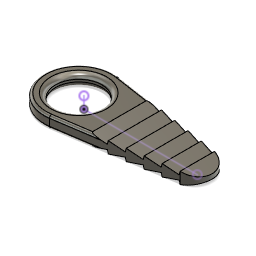
ZugPropfen (Autodesk Fusion 360 design; units mm, degrees)
Autodesk Fusion 360 part; units mm, degrees
sketch "Skizze1" plane through (0, 0, 0) normal (0, 1, 0) x (1, 0, 0)
  circle A0 centre (0, 0) radius 10
  circle A1 centre (0, 0) radius 15
  circle A2 centre (50, 0) radius 7.5
  line L0 (2.25, 14.8303) -> (51.125, 7.4151)
  line L1 (51.125, -7.4151) -> (2.25, -14.8303)
  dimension "d1" = 20
  dimension "d2" = 5
  dimension "d3" = 15
  dimension "d5" = 50
  constraint coincident A0.centre A1.centre
  constraint concentric A0 A1
  constraint coincident A1 L0.start
  constraint coincident A2 L0.end
  constraint tangent A2 L0
  constraint coincident A2 L1.start
  constraint coincident A1 L1.end
  constraint tangent A1 L1
  constraint tangent A1 L0
  constraint tangent A2 L1
  constraint horizontal A0.centre A2.centre
  measures "d1" diameter of A0
  measures "d2" distance of A0 A1
  measures "d3" diameter of A2
  measures "d5" distance of A0.centre A2.centre
extrude "Extrusion1" add sketch "Skizze1" along normal mid plane 5
sketch "Skizze2" plane through (0, 0, 0) normal (0, 0, 1) x (1, 0, 0)
  line L0 (2.25, 2.5) -> (2.25, -2.5)
  line L1 (2.25, -2.5) -> (51.125, -2.5)
sketch "Skizze3" plane through (0, 0, 0) normal (0, 0, 1) x (1, 0, 0)
  line L0 (17.5, 2.5) -> (57.5, 2.5)
  line L1 (57.5, 2.5) -> (57.5, 1)
  line L2 (57.5, 1) -> (51.1276, 2.5)
  line L3 (51.1276, 2.5) -> (50.7745, 1)
  line L4 (50.7745, 1) -> (44.4021, 2.5)
  line L5 (44.4021, 2.5) -> (44.049, 1)
  line L6 (44.049, 1) -> (37.6765, 2.5)
  line L7 (37.6765, 2.5) -> (37.3235, 1)
  line L8 (37.3235, 1) -> (30.951, 2.5)
  line L9 (30.951, 2.5) -> (30.5979, 1)
  line L10 (30.5979, 1) -> (24.2255, 2.5)
  line L11 (24.2255, 2.5) -> (23.8724, 1)
  line L12 (23.8724, 1) -> (17.5, 2.5)
  line L13 (23.8724, 1) -> (57.5, 1) construction
  line L14 (24.2255, 2.5) -> (51.1276, 2.5) construction
  line L15 (51.125, -2.5) -> (51.125, 2.5)
  line L16 (2.25, 2.5) -> (51.125, 2.5)
  line L17 (1.75, 0) -> (22.5, 0)
  line L18 (44.049, -1) -> (37.6765, -2.5)
  line L19 (23.8724, -1) -> (17.5, -2.5)
  line L20 (17.5, -2.5) -> (57.5, -2.5)
  line L21 (24.2255, -2.5) -> (23.8724, -1)
  line L22 (30.951, -2.5) -> (30.5979, -1)
  line L23 (51.1276, -2.5) -> (50.7745, -1)
  line L24 (37.3235, -1) -> (30.951, -2.5)
  line L25 (23.8724, -1) -> (57.5, -1) construction
  line L26 (24.2255, -2.5) -> (51.1276, -2.5) construction
  line L27 (57.5, -2.5) -> (57.5, -1)
  line L28 (37.6765, -2.5) -> (37.3235, -1)
  line L29 (57.5, -1) -> (51.1276, -2.5)
  line L30 (50.7745, -1) -> (44.4021, -2.5)
  line L31 (44.4021, -2.5) -> (44.049, -1)
  line L32 (30.5979, -1) -> (24.2255, -2.5)
  line L33 (51.125, -2.5) -> (51.125, 2.5)
  line L34 (57.5, 2.5) -> (51.125, 2.5)
  line L35 (51.125, 2.5) -> (51.125, -2.5)
  line L36 (51.125, -2.5) -> (57.5, -2.5)
  point P0 (51.125, -2.5)
  dimension "d10" = 40
  dimension "d11" = 1.5
  constraint horizontal L0
  constraint perpendicular L0 L1
  constraint perpendicular L6 L7
  constraint perpendicular L6 L9
  constraint perpendicular L10 L11
  constraint horizontal L13
  constraint coincident L9.end L13
  constraint coincident L7.end L13
  constraint coincident L5.end L13
  constraint coincident L3.end L13
  constraint coincident L8.end L14
  constraint coincident L6.end L14
  constraint coincident L4.end L14
  constraint perpendicular L4 L5
  constraint perpendicular L2 L3
  constraint parallel L10 L12
  constraint parallel L8 L10
  constraint parallel L6 L8
  constraint parallel L4 L6
  constraint parallel L2 L4
  constraint equal L8 L10
  constraint collinear L0 L16
  constraint symmetric L0.start L17 L19.end
  constraint symmetric L0.end L17 L20.end
  constraint symmetric L1.end L17 L25.end
  constraint symmetric L2.end L17 L23.start
  constraint symmetric L3.end L17 L23.end
  constraint symmetric L4.end L17 L30.end
  constraint symmetric L5.end L17 L18.start
  constraint symmetric L6.end L17 L18.end
  constraint symmetric L7.end L17 L24.start
  constraint symmetric L8.end L17 L22.start
  constraint symmetric L9.end L17 L22.end
  constraint symmetric L10.end L17 L21.start
  constraint symmetric L11.end L17 L19.start
  constraint symmetric L15.end L17 P0
  constraint coincident L1 L0.end
  constraint collinear L0 L14
  measures "d10" distance of L0.start L0.end
  measures "d11" distance of L0 L13
extrude "Extrusion2" cut sketch "Skizze3" along normal mid plane 30 contours L0 L1 L2 L34 | L0 L3 L4 L15 L16 L33 L35 | L0 L5 L6 L16 | L0 L7 L8 L16 | L0 L9 L10 L16 | L0 L11 L12 L16 | L15 L20 L23 L30 L33 L35 | L19 L20 L21 | L20 L22 L32 | L20 L24 L28 | L18 L20 L31 | L20 L27 L29 L36
fillet "Abrundung1" radius 2 2 edges at (-9.3233, 2.5, -3.6162) (-9.3233, -2.5, 3.6162)
fillet "Abrundung2" radius 1 6 edges at (9.875, 2.5, -13.6735) (-15, 2.5, 0) (9.875, 2.5, 13.6735) (9.875, -2.5, 13.6735) (-15, -2.5, 0) (9.875, -2.5, -13.6735)
